Autodesk Fusion 360 part; units mm, degrees
(part 4 of 5)
sketch "Reset guide collar profile" plane through (0, 0, -12.5) normal (0, 0, 1) x (1, 0, 0) in component "05 Rear electronics housing"
  line L0 (116.2, 51) -> (117.8, 51)
  line L1 (117.8, 51) -> (117.8, 57.2)
  line L2 (117.8, 57.2) -> (116.2, 57.2)
  line L3 (116.2, 57.2) -> (116.2, 51)
  dimension "d865" = 1.6
  dimension "d866" = 6.2
  measures "d865" horizontal distance of L0.start L0.end
  measures "d866" vertical distance of L0.end L1.end
extrude "Reset guide collar" add sketch "Reset guide collar profile" against normal blind 5.3 separate body makes body 101 in component "05 Rear electronics housing"
ref_plane "WorkPlane58" through (0, 51, 0) normal (0, 1, 0) x (0, 0, 1) in component "05 Rear electronics housing"
sketch "Reset collar underside gusset" plane through (0, 51, 0) normal (0, 1, 0) x (1, 0, 0) in component "05 Rear electronics housing"
  line L0 (116.2, 17.8) -> (117.8, 17.8)
  line L1 (117.8, 17.8) -> (117.8, 19.4)
  line L2 (117.8, 19.4) -> (116.2, 17.8)
extrude "Reset collar underside gusset (1)" add sketch "Reset collar underside gusset" along normal blind 6.2 separate body makes body 102 in component "05 Rear electronics housing"
ref_plane "WorkPlane59" through (0, 0, -15.65) normal (0, 0, 1) x (1, 0, 0) in component "05 Rear electronics housing"
sketch "Reset stop root profile" plane through (0, 0, -15.65) normal (0, 0, 1) x (1, 0, 0) in component "05 Rear electronics housing"
  line L0 (114.2, 50.6) -> (117.8, 50.6)
  line L1 (117.8, 50.6) -> (117.8, 51.6)
  line L2 (117.8, 51.6) -> (114.2, 51.6)
  line L3 (114.2, 51.6) -> (114.2, 50.6)
  dimension "d875" = 3.6
  dimension "d876" = 1
  measures "d875" horizontal distance of L0.start L0.end
  measures "d876" vertical distance of L0.end L1.end
extrude "Reset stop root" add sketch "Reset stop root profile" against normal blind 1.75 separate body makes body 103 in component "05 Rear electronics housing"
ref_plane "WorkPlane60" through (0, 50.6, 0) normal (0, 1, 0) x (0, 0, 1) in component "05 Rear electronics housing"
sketch "Reset stop root gusset" plane through (0, 50.6, 0) normal (0, 1, 0) x (1, 0, 0) in component "05 Rear electronics housing"
  line L0 (114.2, 17.4) -> (117.8, 17.4)
  line L1 (117.8, 17.4) -> (117.8, 21)
  line L2 (117.8, 21) -> (114.2, 17.4)
extrude "Reset stop root gusset (1)" add sketch "Reset stop root gusset" along normal blind 1 separate body makes body 104 in component "05 Rear electronics housing"
ref_plane "WorkPlane61" through (0, 0, -15.65) normal (0, 0, 1) x (1, 0, 0) in component "05 Rear electronics housing"
sketch "Reset inward stop profile" plane through (0, 0, -15.65) normal (0, 0, 1) x (1, 0, 0) in component "05 Rear electronics housing"
  line L0 (114.2, 51.6) -> (114.7, 51.6)
  line L1 (114.7, 51.6) -> (114.7, 53.2)
  line L2 (114.7, 53.2) -> (114.2, 53.2)
  line L3 (114.2, 53.2) -> (114.2, 51.6)
  dimension "d885" = 0.5
  dimension "d886" = 1.6
  measures "d885" horizontal distance of L0.start L0.end
  measures "d886" vertical distance of L0.end L1.end
extrude "Reset inward stop" add sketch "Reset inward stop profile" against normal blind 1.75 separate body makes body 105 in component "05 Rear electronics housing"
combine "Union manufactured solid (8)" operation add target body 66 tool bodies 101 102 103 104 105 in component "05 Rear electronics housing"
ref_plane "WorkPlane62" through (0, 57.4, 0) normal (0, 1, 0) x (0, 0, 1) in component "05 Rear electronics housing"
sketch "Charger USB access" plane through (0, 57.4, 0) normal (0, 1, 0) x (1, 0, 0) in component "05 Rear electronics housing"
  line L0 (14.8, 26.2) -> (28.2, 26.2)
  line L1 (28.2, 26.2) -> (28.2, 20.5)
  line L2 (28.2, 20.5) -> (26.2, 18.5)
  line L3 (26.2, 18.5) -> (16.8, 18.5)
  line L4 (16.8, 18.5) -> (14.8, 20.5)
  line L5 (14.8, 20.5) -> (14.8, 26.2)
extrude "Charger USB access (1)" cut sketch "Charger USB access" along normal blind 2.8 bodies 66 in component "05 Rear electronics housing"
ref_plane "WorkPlane63" through (0, 57.4, 0) normal (0, 1, 0) x (0, 0, 1) in component "05 Rear electronics housing"
sketch "XIAO USB access" plane through (0, 57.4, 0) normal (0, 1, 0) x (1, 0, 0) in component "05 Rear electronics housing"
  line L0 (110.4, 28) -> (117.5, 28)
  line L1 (117.5, 28) -> (117.5, 18)
  line L2 (117.5, 18) -> (116, 16.5)
  line L3 (116, 16.5) -> (111.9, 16.5)
  line L4 (111.9, 16.5) -> (110.4, 18)
  line L5 (110.4, 18) -> (110.4, 28)
extrude "XIAO USB access (1)" cut sketch "XIAO USB access" along normal blind 2.8 bodies 66 in component "05 Rear electronics housing"
ref_plane "WorkPlane64" through (0, 57.4, 0) normal (0, 1, 0) x (0, 0, 1) in component "05 Rear electronics housing"
sketch "Power grip insertion and travel" plane through (0, 57.4, 0) normal (0, 1, 0) x (1, 0, 0) in component "05 Rear electronics housing"
  line L0 (55.25, 24.1) -> (64.75, 24.1)
  line L1 (64.75, 24.1) -> (64.75, 21.1)
  line L2 (64.75, 21.1) -> (62.75, 19.1)
  line L3 (62.75, 19.1) -> (57.25, 19.1)
  line L4 (57.25, 19.1) -> (55.25, 21.1)
  line L5 (55.25, 21.1) -> (55.25, 24.1)
extrude "Power grip insertion and travel (1)" cut sketch "Power grip insertion and travel" along normal blind 2.8 bodies 66 in component "05 Rear electronics housing"
ref_plane "WorkPlane65" through (116.1, 0, 0) normal (1, 0, 0) x (0, 1, 0) in component "05 Rear electronics housing"
sketch "Reset stem guide" plane through (116.1, 0, 0) normal (1, 0, 0) x (0, 0, -1) in component "05 Rear electronics housing"
  line L0 (16.6, 52.55) -> (16.6, 56.85)
  line L1 (16.6, 56.85) -> (14, 56.85)
  line L2 (14, 56.85) -> (13.7, 56.55)
  line L3 (13.7, 56.55) -> (13.7, 52.85)
  line L4 (13.7, 52.85) -> (14, 52.55)
  line L5 (14, 52.55) -> (16.6, 52.55)
extrude "Reset stem guide (1)" cut sketch "Reset stem guide" along normal blind 4.1 bodies 66 in component "05 Rear electronics housing"
ref_plane "WorkPlane66" through (0, 0, -15.64) normal (0, 0, 1) x (1, 0, 0) in component "05 Rear electronics housing"
sketch "Open reset insertion path - stop moved to yoke profile" plane through (0, 0, -15.64) normal (0, 0, 1) x (1, 0, 0) in component "05 Rear electronics housing"
  line L0 (114.19, 50.59) -> (116.19, 50.59)
  line L1 (116.19, 50.59) -> (116.19, 53.21)
  line L2 (116.19, 53.21) -> (114.19, 53.21)
  line L3 (114.19, 53.21) -> (114.19, 50.59)
  dimension "d907" = 2
  dimension "d908" = 2.62
  measures "d907" horizontal distance of L0.start L0.end
  measures "d908" vertical distance of L0.end L1.end
extrude "Open reset insertion path - stop moved to yoke" cut sketch "Open reset insertion path - stop moved to yoke profile" against normal blind 5.37 bodies 66 in component "05 Rear electronics housing"
ref_plane "WorkPlane1" through (0, 0, -9.4) normal (0, 0, 1) x (1, 0, 0) in component "06 Electronics retaining yoke"
sketch "Common yoke rail profile" plane through (0, 0, -9.4) normal (0, 0, 1) x (1, 0, 0) in component "06 Electronics retaining yoke"
  line L0 (11.1, 36) -> (112.3, 36)
  line L1 (112.3, 36) -> (112.3, 39)
  line L2 (112.3, 39) -> (11.1, 39)
  line L3 (11.1, 39) -> (11.1, 36)
  dimension "d913" = 101.2
  dimension "d914" = 3
  measures "d913" horizontal distance of L0.start L0.end
  measures "d914" vertical distance of L0.end L1.end
extrude "Common yoke rail" add sketch "Common yoke rail profile" against normal blind 2 separate body makes body 106 in component "06 Electronics retaining yoke"
ref_plane "WorkPlane2" through (0, 0, -9.4) normal (0, 0, 1) x (1, 0, 0) in component "06 Electronics retaining yoke"
sketch "Charger yoke arm profile" plane through (0, 0, -9.4) normal (0, 0, 1) x (1, 0, 0) in component "06 Electronics retaining yoke"
  line L0 (11.1, 34) -> (15.7, 34)
  line L1 (15.7, 34) -> (15.7, 53)
  line L2 (15.7, 53) -> (11.1, 53)
  line L3 (11.1, 53) -> (11.1, 34)
  dimension "d919" = 4.6
  dimension "d920" = 19
  measures "d919" horizontal distance of L0.start L0.end
  measures "d920" vertical distance of L0.end L1.end
extrude "Charger yoke arm" add sketch "Charger yoke arm profile" against normal blind 2 separate body makes body 107 in component "06 Electronics retaining yoke"
ref_plane "WorkPlane3" through (0, 0, -9.4) normal (0, 0, 1) x (1, 0, 0) in component "06 Electronics retaining yoke"
sketch "Charger yoke arm profile (1)" plane through (0, 0, -9.4) normal (0, 0, 1) x (1, 0, 0) in component "06 Electronics retaining yoke"
  line L0 (26.9, 34) -> (31.5, 34)
  line L1 (31.5, 34) -> (31.5, 53)
  line L2 (31.5, 53) -> (26.9, 53)
  line L3 (26.9, 53) -> (26.9, 34)
  dimension "d925" = 4.6
  dimension "d926" = 19
  measures "d925" horizontal distance of L0.start L0.end
  measures "d926" vertical distance of L0.end L1.end
extrude "Charger yoke arm (1)" add sketch "Charger yoke arm profile (1)" against normal blind 2 separate body makes body 108 in component "06 Electronics retaining yoke"
ref_plane "WorkPlane4" through (0, 0, -11.4) normal (0, 0, 1) x (1, 0, 0) in component "06 Electronics retaining yoke"
sketch "Charger keeper foot profile" plane through (0, 0, -11.4) normal (0, 0, 1) x (1, 0, 0) in component "06 Electronics retaining yoke"
  line L0 (13.1, 34) -> (15.1, 34)
  line L1 (15.1, 34) -> (15.1, 36)
  line L2 (15.1, 36) -> (13.1, 36)
  line L3 (13.1, 36) -> (13.1, 34)
  dimension "d931" = 2
  dimension "d932" = 2
  measures "d931" horizontal distance of L0.start L0.end
  measures "d932" vertical distance of L0.end L1.end
extrude "Charger keeper foot" add sketch "Charger keeper foot profile" against normal blind 11.65 separate body makes body 109 in component "06 Electronics retaining yoke"
ref_plane "WorkPlane5" through (0, 0, -11.4) normal (0, 0, 1) x (1, 0, 0) in component "06 Electronics retaining yoke"
sketch "Charger keeper foot profile (1)" plane through (0, 0, -11.4) normal (0, 0, 1) x (1, 0, 0) in component "06 Electronics retaining yoke"
  line L0 (26.9, 34) -> (28.9, 34)
  line L1 (28.9, 34) -> (28.9, 36)
  line L2 (28.9, 36) -> (26.9, 36)
  line L3 (26.9, 36) -> (26.9, 34)
  dimension "d937" = 2
  dimension "d938" = 2
  measures "d937" horizontal distance of L0.start L0.end
  measures "d938" vertical distance of L0.end L1.end
extrude "Charger keeper foot (1)" add sketch "Charger keeper foot profile (1)" against normal blind 11.65 separate body makes body 110 in component "06 Electronics retaining yoke"
ref_plane "WorkPlane6" through (0, 0, -11.4) normal (0, 0, 1) x (1, 0, 0) in component "06 Electronics retaining yoke"
sketch "Charger keeper foot profile (2)" plane through (0, 0, -11.4) normal (0, 0, 1) x (1, 0, 0) in component "06 Electronics retaining yoke"
  line L0 (13.1, 51) -> (15.1, 51)
  line L1 (15.1, 51) -> (15.1, 53)
  line L2 (15.1, 53) -> (13.1, 53)
  line L3 (13.1, 53) -> (13.1, 51)
  dimension "d943" = 2
  dimension "d944" = 2
  measures "d943" horizontal distance of L0.start L0.end
  measures "d944" vertical distance of L0.end L1.end
extrude "Charger keeper foot (2)" add sketch "Charger keeper foot profile (2)" against normal blind 11.65 separate body makes body 111 in component "06 Electronics retaining yoke"
ref_plane "WorkPlane7" through (0, 0, -11.4) normal (0, 0, 1) x (1, 0, 0) in component "06 Electronics retaining yoke"
sketch "Charger keeper foot profile (3)" plane through (0, 0, -11.4) normal (0, 0, 1) x (1, 0, 0) in component "06 Electronics retaining yoke"
  line L0 (26.9, 51) -> (28.9, 51)
  line L1 (28.9, 51) -> (28.9, 53)
  line L2 (28.9, 53) -> (26.9, 53)
  line L3 (26.9, 53) -> (26.9, 51)
  dimension "d949" = 2
  dimension "d950" = 2
  measures "d949" horizontal distance of L0.start L0.end
  measures "d950" vertical distance of L0.end L1.end
extrude "Charger keeper foot (3)" add sketch "Charger keeper foot profile (3)" against normal blind 11.65 separate body makes body 112 in component "06 Electronics retaining yoke"
ref_plane "WorkPlane8" through (0, 0, -9.4) normal (0, 0, 1) x (1, 0, 0) in component "06 Electronics retaining yoke"
sketch "Switch yoke arm profile" plane through (0, 0, -9.4) normal (0, 0, 1) x (1, 0, 0) in component "06 Electronics retaining yoke"
  line L0 (53.5, 37) -> (56.9, 37)
  line L1 (56.9, 37) -> (56.9, 52)
  line L2 (56.9, 52) -> (53.5, 52)
  line L3 (53.5, 52) -> (53.5, 37)
  dimension "d955" = 3.4
  dimension "d956" = 15
  measures "d955" horizontal distance of L0.start L0.end
  measures "d956" vertical distance of L0.end L1.end
extrude "Switch yoke arm" add sketch "Switch yoke arm profile" against normal blind 2 separate body makes body 113 in component "06 Electronics retaining yoke"
ref_plane "WorkPlane9" through (0, 0, -9.4) normal (0, 0, 1) x (1, 0, 0) in component "06 Electronics retaining yoke"
sketch "Switch yoke arm profile (1)" plane through (0, 0, -9.4) normal (0, 0, 1) x (1, 0, 0) in component "06 Electronics retaining yoke"
  line L0 (63.1, 37) -> (66.5, 37)
  line L1 (66.5, 37) -> (66.5, 52)
  line L2 (66.5, 52) -> (63.1, 52)
  line L3 (63.1, 52) -> (63.1, 37)
  dimension "d961" = 3.4
  dimension "d962" = 15
  measures "d961" horizontal distance of L0.start L0.end
  measures "d962" vertical distance of L0.end L1.end
extrude "Switch yoke arm (1)" add sketch "Switch yoke arm profile (1)" against normal blind 2 separate body makes body 114 in component "06 Electronics retaining yoke"
ref_plane "WorkPlane10" through (0, 0, -11.4) normal (0, 0, 1) x (1, 0, 0) in component "06 Electronics retaining yoke"
sketch "Switch retaining foot profile" plane through (0, 0, -11.4) normal (0, 0, 1) x (1, 0, 0) in component "06 Electronics retaining yoke"
  line L0 (55.9, 49.7) -> (56.9, 49.7)
  line L1 (56.9, 49.7) -> (56.9, 52)
  line L2 (56.9, 52) -> (55.9, 52)
  line L3 (55.9, 52) -> (55.9, 49.7)
  dimension "d967" = 1
  dimension "d968" = 2.3
  measures "d967" horizontal distance of L0.start L0.end
  measures "d968" vertical distance of L0.end L1.end
extrude "Switch retaining foot" add sketch "Switch retaining foot profile" against normal blind 8.45 separate body makes body 115 in component "06 Electronics retaining yoke"
ref_plane "WorkPlane11" through (0, 0, -11.4) normal (0, 0, 1) x (1, 0, 0) in component "06 Electronics retaining yoke"
sketch "Switch retaining foot profile (1)" plane through (0, 0, -11.4) normal (0, 0, 1) x (1, 0, 0) in component "06 Electronics retaining yoke"
  line L0 (63.1, 49.7) -> (64.1, 49.7)
  line L1 (64.1, 49.7) -> (64.1, 52)
  line L2 (64.1, 52) -> (63.1, 52)
  line L3 (63.1, 52) -> (63.1, 49.7)
  dimension "d973" = 1
  dimension "d974" = 2.3
  measures "d973" horizontal distance of L0.start L0.end
  measures "d974" vertical distance of L0.end L1.end
extrude "Switch retaining foot (1)" add sketch "Switch retaining foot profile (1)" against normal blind 8.45 separate body makes body 116 in component "06 Electronics retaining yoke"
ref_plane "WorkPlane12" through (0, 0, -9.4) normal (0, 0, 1) x (1, 0, 0) in component "06 Electronics retaining yoke"
sketch "XIAO yoke rail profile" plane through (0, 0, -9.4) normal (0, 0, 1) x (1, 0, 0) in component "06 Electronics retaining yoke"
  line L0 (108.5, 38) -> (112.3, 38)
  line L1 (112.3, 38) -> (112.3, 50)
  line L2 (112.3, 50) -> (108.5, 50)
  line L3 (108.5, 50) -> (108.5, 38)
  dimension "d979" = 3.8
  dimension "d980" = 12
  measures "d979" horizontal distance of L0.start L0.end
  measures "d980" vertical distance of L0.end L1.end
extrude "XIAO yoke rail" add sketch "XIAO yoke rail profile" against normal blind 2 separate body makes body 117 in component "06 Electronics retaining yoke"
ref_plane "WorkPlane13" through (0, 0, -9.4) normal (0, 0, 1) x (1, 0, 0) in component "06 Electronics retaining yoke"
sketch "Reset stop arm profile" plane through (0, 0, -9.4) normal (0, 0, 1) x (1, 0, 0) in component "06 Electronics retaining yoke"
  line L0 (108.5, 49) -> (115.4, 49)
  line L1 (115.4, 49) -> (115.4, 51.6)
  line L2 (115.4, 51.6) -> (108.5, 51.6)
  line L3 (108.5, 51.6) -> (108.5, 49)
  dimension "d985" = 6.9
  dimension "d986" = 2.6
  measures "d985" horizontal distance of L0.start L0.end
  measures "d986" vertical distance of L0.end L1.end
extrude "Reset stop arm" add sketch "Reset stop arm profile" against normal blind 2 separate body makes body 118 in component "06 Electronics retaining yoke"
ref_plane "WorkPlane14" through (0, 0, -11.4) normal (0, 0, 1) x (1, 0, 0) in component "06 Electronics retaining yoke"
sketch "Reset stop post profile" plane through (0, 0, -11.4) normal (0, 0, 1) x (1, 0, 0) in component "06 Electronics retaining yoke"
  line L0 (113.5, 50.6) -> (115.4, 50.6)
  line L1 (115.4, 50.6) -> (115.4, 51.6)
  line L2 (115.4, 51.6) -> (113.5, 51.6)
  line L3 (113.5, 51.6) -> (113.5, 50.6)
  dimension "d991" = 1.9
  dimension "d992" = 1
  measures "d991" horizontal distance of L0.start L0.end
  measures "d992" vertical distance of L0.end L1.end
extrude "Reset stop post" add sketch "Reset stop post profile" against normal blind 6 separate body makes body 119 in component "06 Electronics retaining yoke"
ref_plane "WorkPlane15" through (0, 0, -15.65) normal (0, 0, 1) x (1, 0, 0) in component "06 Electronics retaining yoke"
sketch "Reset inward stop profile (2)" plane through (0, 0, -15.65) normal (0, 0, 1) x (1, 0, 0) in component "06 Electronics retaining yoke"
  line L0 (113.5, 51.6) -> (114.7, 51.6)
  line L1 (114.7, 51.6) -> (114.7, 53.2)
  line L2 (114.7, 53.2) -> (113.5, 53.2)
  line L3 (113.5, 53.2) -> (113.5, 51.6)
  dimension "d997" = 1.2
  dimension "d998" = 1.6
  measures "d997" horizontal distance of L0.start L0.end
  measures "d998" vertical distance of L0.end L1.end
extrude "Reset inward stop'" add sketch "Reset inward stop profile (2)" against normal blind 1.75 separate body makes body 120 in component "06 Electronics retaining yoke"
ref_plane "WorkPlane16" through (113.5, 0, 0) normal (1, 0, 0) x (0, 1, 0) in component "06 Electronics retaining yoke"
sketch "Reset stop 45 degree brace" plane through (113.5, 0, 0) normal (1, 0, 0) x (0, 0, -1) in component "06 Electronics retaining yoke"
  line L0 (14.05, 51.6) -> (15.65, 51.6)
  line L1 (15.65, 51.6) -> (15.65, 53.2)
  line L2 (15.65, 53.2) -> (14.05, 51.6)
extrude "Reset stop 45 degree brace (1)" add sketch "Reset stop 45 degree brace" along normal blind 1.2 separate body makes body 121 in component "06 Electronics retaining yoke"
ref_plane "WorkPlane17" through (0, 0, -9.4) normal (0, 0, 1) x (1, 0, 0) in component "06 Electronics retaining yoke"
sketch "XIAO restraint root profile" plane through (0, 0, -9.4) normal (0, 0, 1) x (1, 0, 0) in component "06 Electronics retaining yoke"
  line L0 (111.8, 40) -> (113.75, 40)
  line L1 (113.75, 40) -> (113.75, 42)
  line L2 (113.75, 42) -> (111.8, 42)
  line L3 (111.8, 42) -> (111.8, 40)
  dimension "d1007" = 1.95
  dimension "d1008" = 2
  measures "d1007" horizontal distance of L0.start L0.end
  measures "d1008" vertical distance of L0.end L1.end
extrude "XIAO restraint root" add sketch "XIAO restraint root profile" against normal blind 2 separate body makes body 122 in component "06 Electronics retaining yoke"
ref_plane "WorkPlane18" through (0, 0, -11.3) normal (0, 0, 1) x (1, 0, 0) in component "06 Electronics retaining yoke"
sketch "XIAO front outer restraint profile" plane through (0, 0, -11.3) normal (0, 0, 1) x (1, 0, 0) in component "06 Electronics retaining yoke"
  line L0 (112.25, 40) -> (113.75, 40)
  line L1 (113.75, 40) -> (113.75, 42)
  line L2 (113.75, 42) -> (112.25, 42)
  line L3 (112.25, 42) -> (112.25, 40)
  dimension "d1013" = 1.5
  dimension "d1014" = 2
  measures "d1013" horizontal distance of L0.start L0.end
  measures "d1014" vertical distance of L0.end L1.end
extrude "XIAO front outer restraint" add sketch "XIAO front outer restraint profile" against normal blind 2.4 separate body makes body 123 in component "06 Electronics retaining yoke"
ref_plane "WorkPlane19" through (0, 0, -9.4) normal (0, 0, 1) x (1, 0, 0) in component "06 Electronics retaining yoke"
sketch "XIAO restraint root profile (1)" plane through (0, 0, -9.4) normal (0, 0, 1) x (1, 0, 0) in component "06 Electronics retaining yoke"
  line L0 (111.8, 48) -> (113.75, 48)
  line L1 (113.75, 48) -> (113.75, 50)
  line L2 (113.75, 50) -> (111.8, 50)
  line L3 (111.8, 50) -> (111.8, 48)
  dimension "d1019" = 1.95
  dimension "d1020" = 2
  measures "d1019" horizontal distance of L0.start L0.end
  measures "d1020" vertical distance of L0.end L1.end
extrude "XIAO restraint root (1)" add sketch "XIAO restraint root profile (1)" against normal blind 2 separate body makes body 124 in component "06 Electronics retaining yoke"
ref_plane "WorkPlane20" through (0, 0, -11.3) normal (0, 0, 1) x (1, 0, 0) in component "06 Electronics retaining yoke"
sketch "XIAO front outer restraint profile (1)" plane through (0, 0, -11.3) normal (0, 0, 1) x (1, 0, 0) in component "06 Electronics retaining yoke"
  line L0 (112.25, 48) -> (113.75, 48)
  line L1 (113.75, 48) -> (113.75, 50)
  line L2 (113.75, 50) -> (112.25, 50)
  line L3 (112.25, 50) -> (112.25, 48)
  dimension "d1025" = 1.5
  dimension "d1026" = 2
  measures "d1025" horizontal distance of L0.start L0.end
  measures "d1026" vertical distance of L0.end L1.end
extrude "XIAO front outer restraint (1)" add sketch "XIAO front outer restraint profile (1)" against normal blind 2.4 separate body makes body 125 in component "06 Electronics retaining yoke"
ref_plane "WorkPlane21" through (0, 0, -9.4) normal (0, 0, 1) x (1, 0, 0) in component "06 Electronics retaining yoke"
sketch "Yoke screw pad profile" plane through (0, 0, -9.4) normal (0, 0, 1) x (1, 0, 0) in component "06 Electronics retaining yoke"
  line L0 (30.8, 33.8) -> (39.2, 33.8)
  line L1 (39.2, 33.8) -> (39.2, 42.2)
  line L2 (39.2, 42.2) -> (30.8, 42.2)
  line L3 (30.8, 42.2) -> (30.8, 33.8)
  dimension "d1031" = 8.4
  dimension "d1032" = 8.4
  measures "d1031" horizontal distance of L0.start L0.end
  measures "d1032" vertical distance of L0.end L1.end
extrude "Yoke screw pad" add sketch "Yoke screw pad profile" against normal blind 2 separate body makes body 126 in component "06 Electronics retaining yoke"
ref_plane "WorkPlane22" through (0, 0, -9.4) normal (0, 0, 1) x (1, 0, 0) in component "06 Electronics retaining yoke"
sketch "Yoke screw pad profile (1)" plane through (0, 0, -9.4) normal (0, 0, 1) x (1, 0, 0) in component "06 Electronics retaining yoke"
  line L0 (98.8, 33.8) -> (107.2, 33.8)
  line L1 (107.2, 33.8) -> (107.2, 42.2)
  line L2 (107.2, 42.2) -> (98.8, 42.2)
  line L3 (98.8, 42.2) -> (98.8, 33.8)
  dimension "d1037" = 8.4
  dimension "d1038" = 8.4
  measures "d1037" horizontal distance of L0.start L0.end
  measures "d1038" vertical distance of L0.end L1.end
extrude "Yoke screw pad (1)" add sketch "Yoke screw pad profile (1)" against normal blind 2 separate body makes body 127 in component "06 Electronics retaining yoke"
combine "Union manufactured solid''''" operation add target body 106 tool bodies 107 108 109 110 111 112 113 114 115 116 117 118 119 120 121 122 123 124 125 126 127 in component "06 Electronics retaining yoke"
ref_plane "WorkPlane23" through (0, 0, -9.38) normal (0, 0, 1) x (1, 0, 0) in component "06 Electronics retaining yoke"
sketch "Yoke M3 clearance profile" plane through (0, 0, -9.38) normal (0, 0, 1) x (1, 0, 0) in component "06 Electronics retaining yoke"
  circle A0 centre (35, 38) radius 1.7
  dimension "d1043" = 3.4
  measures "d1043" diameter of A0
extrude "Yoke M3 clearance" cut sketch "Yoke M3 clearance profile" against normal blind 2.04 bodies 106 in component "06 Electronics retaining yoke"
ref_plane "WorkPlane24" through (0, 0, -9.38) normal (0, 0, 1) x (1, 0, 0) in component "06 Electronics retaining yoke"
sketch "Yoke M3 clearance profile (1)" plane through (0, 0, -9.38) normal (0, 0, 1) x (1, 0, 0) in component "06 Electronics retaining yoke"
  circle A0 centre (103, 38) radius 1.7
  dimension "d1048" = 3.4
  measures "d1048" diameter of A0
extrude "Yoke M3 clearance (1)" cut sketch "Yoke M3 clearance profile (1)" against normal blind 2.04 bodies 106 in component "06 Electronics retaining yoke"
ref_plane "WorkPlane1" through (0, 0, -13.95) normal (0, 0, 1) x (1, 0, 0) in component "07 Captive reset plunger"
sketch "Reset exterior stem profile" plane through (0, 0, -13.95) normal (0, 0, 1) x (1, 0, 0) in component "07 Captive reset plunger"
  line L0 (116, 52.8) -> (120.6, 52.8)
  line L1 (120.6, 52.8) -> (120.6, 56.6)
  line L2 (120.6, 56.6) -> (116, 56.6)
  line L3 (116, 56.6) -> (116, 52.8)
  dimension "d1053" = 4.6
  dimension "d1054" = 3.8
  measures "d1053" horizontal distance of L0.start L0.end
  measures "d1054" vertical distance of L0.end L1.end
extrude "Reset exterior stem" add sketch "Reset exterior stem profile" against normal blind 2.4 separate body makes body 128 in component "07 Captive reset plunger"
ref_plane "WorkPlane2" through (0, 0, -13.95) normal (0, 0, 1) x (1, 0, 0) in component "07 Captive reset plunger"
sketch "Reset captive flange profile" plane through (0, 0, -13.95) normal (0, 0, 1) x (1, 0, 0) in component "07 Captive reset plunger"
  line L0 (115.2, 51.9) -> (116, 51.9)
  line L1 (116, 51.9) -> (116, 57.5)
  line L2 (116, 57.5) -> (115.2, 57.5)
  line L3 (115.2, 57.5) -> (115.2, 51.9)
  dimension "d1059" = 0.8
  dimension "d1060" = 5.6
  measures "d1059" horizontal distance of L0.start L0.end
  measures "d1060" vertical distance of L0.end L1.end
extrude "Reset captive flange" add sketch "Reset captive flange profile" against normal blind 3.2 separate body makes body 129 in component "07 Captive reset plunger"
ref_plane "WorkPlane3" through (0, 0, -13.95) normal (0, 0, 1) x (1, 0, 0) in component "07 Captive reset plunger"
sketch "Reset contact tip profile" plane through (0, 0, -13.95) normal (0, 0, 1) x (1, 0, 0) in component "07 Captive reset plunger"
  line L0 (113.7, 53.9) -> (115.2, 53.9)
  line L1 (115.2, 53.9) -> (115.2, 55.5)
  line L2 (115.2, 55.5) -> (113.7, 55.5)
  line L3 (113.7, 55.5) -> (113.7, 53.9)
  dimension "d1065" = 1.5
  dimension "d1066" = 1.6
  measures "d1065" horizontal distance of L0.start L0.end
  measures "d1066" vertical distance of L0.end L1.end
extrude "Reset contact tip" add sketch "Reset contact tip profile" against normal blind 1.2 separate body makes body 130 in component "07 Captive reset plunger"
combine "Union manufactured solid'''''" operation add target body 128 tool bodies 129 130 in component "07 Captive reset plunger"
ref_plane "WorkPlane1" through (0, 0, -20.05) normal (0, 0, 1) x (1, 0, 0) in component "08 Captive DPDT power slider"
sketch "Actuator cup blank profile" plane through (0, 0, -20.05) normal (0, 0, 1) x (1, 0, 0) in component "08 Captive DPDT power slider"
  line L0 (57.7, 52.4) -> (62.3, 52.4)
  line L1 (62.3, 52.4) -> (62.3, 53.4)
  line L2 (62.3, 53.4) -> (57.7, 53.4)
  line L3 (57.7, 53.4) -> (57.7, 52.4)
  dimension "d1071" = 4.6
  dimension "d1072" = 1
  measures "d1071" horizontal distance of L0.start L0.end
  measures "d1072" vertical distance of L0.end L1.end
extrude "Actuator cup blank" add sketch "Actuator cup blank profile" against normal blind 3.3 separate body makes body 131 in component "08 Captive DPDT power slider"
ref_plane "WorkPlane2" through (0, 53.4, 0) normal (0, 1, 0) x (0, 0, 1) in component "08 Captive DPDT power slider"
sketch "Slider shoulder lower" plane through (0, 53.4, 0) normal (0, 1, 0) x (1, 0, 0) in component "08 Captive DPDT power slider"
  line L0 (57.7, 20.05) -> (62.3, 20.05)
  line L1 (62.3, 20.05) -> (62.3, 23.35)
  line L2 (62.3, 23.35) -> (57.7, 23.35)
  line L3 (57.7, 23.35) -> (57.7, 20.05)
ref_plane "WorkPlane3" through (0, 57.1, 0) normal (0, 1, 0) x (0, 0, 1) in component "08 Captive DPDT power slider"
sketch "Slider shoulder upper" plane through (0, 57.1, 0) normal (0, 1, 0) x (1, 0, 0) in component "08 Captive DPDT power slider"
  line L0 (54, 18.5) -> (66, 18.5)
  line L1 (66, 18.5) -> (66, 25.5)
  line L2 (66, 25.5) -> (54, 25.5)
  line L3 (54, 25.5) -> (54, 18.5)
loft "Self-supporting slider shoulder" add profiles "Slider shoulder lower", "Slider shoulder upper" section 1 section 2 separate body makes body 132 in component "08 Captive DPDT power slider"
ref_plane "WorkPlane4" through (0, 0, -18.5) normal (0, 0, 1) x (1, 0, 0) in component "08 Captive DPDT power slider"
sketch "Inner captive flange profile" plane through (0, 0, -18.5) normal (0, 0, 1) x (1, 0, 0) in component "08 Captive DPDT power slider"
  line L0 (54, 57.05) -> (66, 57.05)
  line L1 (66, 57.05) -> (66, 57.4)
  line L2 (66, 57.4) -> (54, 57.4)
  line L3 (54, 57.4) -> (54, 57.05)
  dimension "d1081" = 12
  dimension "d1082" = 0.35
  measures "d1081" horizontal distance of L0.start L0.end
  measures "d1082" vertical distance of L0.end L1.end
extrude "Inner captive flange" add sketch "Inner captive flange profile" against normal blind 7 separate body makes body 133 in component "08 Captive DPDT power slider"
ref_plane "WorkPlane5" through (0, 0, -20.8) normal (0, 0, 1) x (1, 0, 0) in component "08 Captive DPDT power slider"
sketch "Slider guide neck profile" plane through (0, 0, -20.8) normal (0, 0, 1) x (1, 0, 0) in component "08 Captive DPDT power slider"
  line L0 (57.6, 57.3) -> (62.4, 57.3)
  line L1 (62.4, 57.3) -> (62.4, 60.8)
  line L2 (62.4, 60.8) -> (57.6, 60.8)
  line L3 (57.6, 60.8) -> (57.6, 57.3)
  dimension "d1087" = 4.8
  dimension "d1088" = 3.5
  measures "d1087" horizontal distance of L0.start L0.end
  measures "d1088" vertical distance of L0.end L1.end
extrude "Slider guide neck" add sketch "Slider guide neck profile" against normal blind 2.4 separate body makes body 134 in component "08 Captive DPDT power slider"
ref_plane "WorkPlane6" through (0, 0, -20.6) normal (0, 0, 1) x (1, 0, 0) in component "08 Captive DPDT power slider"
sketch "Exterior finger grip profile" plane through (0, 0, -20.6) normal (0, 0, 1) x (1, 0, 0) in component "08 Captive DPDT power slider"
  line L0 (57.5, 60) -> (62.5, 60)
  line L1 (62.5, 60) -> (62.5, 61.4)
  line L2 (62.5, 61.4) -> (57.5, 61.4)
  line L3 (57.5, 61.4) -> (57.5, 60)
  dimension "d1093" = 5
  dimension "d1094" = 1.4
  measures "d1093" horizontal distance of L0.start L0.end
  measures "d1094" vertical distance of L0.end L1.end
extrude "Exterior finger grip" add sketch "Exterior finger grip profile" against normal blind 2.8 separate body makes body 135 in component "08 Captive DPDT power slider"
combine "Union manufactured solid''''''" operation add target body 131 tool bodies 132 133 134 135 in component "08 Captive DPDT power slider"
ref_plane "WorkPlane7" through (0, 0, -18) normal (0, 0, 1) x (1, 0, 0) in component "08 Captive DPDT power slider"
sketch "Front and bottom open actuator fork profile" plane through (0, 0, -18) normal (0, 0, 1) x (1, 0, 0) in component "08 Captive DPDT power slider"
  line L0 (59.09, 52.3) -> (60.91, 52.3)
  line L1 (60.91, 52.3) -> (60.91, 54.43)
  line L2 (60.91, 54.43) -> (59.09, 54.43)
  line L3 (59.09, 54.43) -> (59.09, 52.3)
  dimension "d1099" = 1.82
  dimension "d1100" = 2.13
  measures "d1099" horizontal distance of L0.start L0.end
  measures "d1100" vertical distance of L0.end L1.end
extrude "Front and bottom open actuator fork" cut sketch "Front and bottom open actuator fork profile" against normal blind 4.46 bodies 131 in component "08 Captive DPDT power slider"
ref_plane "WorkPlane1" through (0, 0, -20.6) normal (0, 0, 1) x (1, 0, 0) in component "REF Battery"
sketch "Battery pouch profile" plane through (0, 0, -20.6) normal (0, 0, 1) x (1, 0, 0) in component "REF Battery"
  line L0 (35, 11) -> (87, 11)
  line L1 (87, 11) -> (87, 32)
  line L2 (87, 32) -> (35, 32)
  line L3 (35, 32) -> (35, 11)
  dimension "d1105" = 52
  dimension "d1106" = 21
  measures "d1105" horizontal distance of L0.start L0.end
  measures "d1106" vertical distance of L0.end L1.end
extrude "Battery pouch" add sketch "Battery pouch profile" against normal blind 10 separate body makes body 136 in component "REF Battery"
ref_plane "WorkPlane1" through (0, 0, -23.2) normal (0, 0, 1) x (1, 0, 0) in component "REF Charger"
sketch "Charger PCB profile" plane through (0, 0, -23.2) normal (0, 0, 1) x (1, 0, 0) in component "REF Charger"
  line L0 (12.75, 32) -> (29.25, 32)
  line L1 (29.25, 32) -> (29.25, 57)
  line L2 (29.25, 57) -> (12.75, 57)
  line L3 (12.75, 57) -> (12.75, 32)
  dimension "d1111" = 16.5
  dimension "d1112" = 25
  measures "d1111" horizontal distance of L0.start L0.end
  measures "d1112" vertical distance of L0.end L1.end
extrude "Charger PCB" add sketch "Charger PCB profile" against normal blind 1 separate body makes body 137 in component "REF Charger"
ref_plane "WorkPlane2" through (0, 0, -19.6) normal (0, 0, 1) x (1, 0, 0) in component "REF Charger"
sketch "Charger USB envelope profile" plane through (0, 0, -19.6) normal (0, 0, 1) x (1, 0, 0) in component "REF Charger"
  line L0 (17, 53) -> (26, 53)
  line L1 (26, 53) -> (26, 59.4)
  line L2 (26, 59.4) -> (17, 59.4)
  line L3 (17, 59.4) -> (17, 53)
  dimension "d1117" = 9
  dimension "d1118" = 6.4
  measures "d1117" horizontal distance of L0.start L0.end
  measures "d1118" vertical distance of L0.end L1.end
extrude "Charger USB envelope" add sketch "Charger USB envelope profile" against normal blind 3.6 separate body makes body 138 in component "REF Charger"
ref_plane "WorkPlane3" through (0, 0, -20.9) normal (0, 0, 1) x (1, 0, 0) in component "REF Charger"
sketch "Charger IC envelope profile" plane through (0, 0, -20.9) normal (0, 0, 1) x (1, 0, 0) in component "REF Charger"
  line L0 (18, 36) -> (25, 36)
  line L1 (25, 36) -> (25, 47)
  line L2 (25, 47) -> (18, 47)
  line L3 (18, 47) -> (18, 36)
  dimension "d1123" = 7
  dimension "d1124" = 11
  measures "d1123" horizontal distance of L0.start L0.end
  measures "d1124" vertical distance of L0.end L1.end
extrude "Charger IC envelope" add sketch "Charger IC envelope profile" against normal blind 2.3 separate body makes body 139 in component "REF Charger"
ref_plane "WorkPlane1" through (0, 0, -11.55) normal (0, 0, 1) x (1, 0, 0) in component "REF XIAO"
sketch "XIAO PCB profile" plane through (0, 0, -11.55) normal (0, 0, 1) x (1, 0, 0) in component "REF XIAO"
  line L0 (111, 35.5) -> (112, 35.5)
  line L1 (112, 35.5) -> (112, 56.5)
  line L2 (112, 56.5) -> (111, 56.5)
  line L3 (111, 56.5) -> (111, 35.5)
  dimension "d1129" = 1
  dimension "d1130" = 21
  measures "d1129" horizontal distance of L0.start L0.end
  measures "d1130" vertical distance of L0.end L1.end
extrude "XIAO PCB" add sketch "XIAO PCB profile" against normal blind 17.8 separate body makes body 140 in component "REF XIAO"
ref_plane "WorkPlane2" through (0, 0, -17.75) normal (0, 0, 1) x (1, 0, 0) in component "REF XIAO"
sketch "XIAO USB envelope profile" plane through (0, 0, -17.75) normal (0, 0, 1) x (1, 0, 0) in component "REF XIAO"
  line L0 (112, 52) -> (115.3, 52)
  line L1 (115.3, 52) -> (115.3, 58.4)
  line L2 (115.3, 58.4) -> (112, 58.4)
  line L3 (112, 58.4) -> (112, 52)
  dimension "d1135" = 3.3
  dimension "d1136" = 6.4
  measures "d1135" horizontal distance of L0.start L0.end
  measures "d1136" vertical distance of L0.end L1.end
extrude "XIAO USB envelope" add sketch "XIAO USB envelope profile" against normal blind 9 separate body makes body 141 in component "REF XIAO"
ref_plane "WorkPlane3" through (0, 0, -16) normal (0, 0, 1) x (1, 0, 0) in component "REF XIAO"
sketch "XIAO component envelope profile" plane through (0, 0, -16) normal (0, 0, 1) x (1, 0, 0) in component "REF XIAO"
  line L0 (112, 41.5) -> (115, 41.5)
  line L1 (115, 41.5) -> (115, 50.5)
  line L2 (115, 50.5) -> (112, 50.5)
  line L3 (112, 50.5) -> (112, 41.5)
  dimension "d1141" = 3
  dimension "d1142" = 9
  measures "d1141" horizontal distance of L0.start L0.end
  measures "d1142" vertical distance of L0.end L1.end
extrude "XIAO component envelope" add sketch "XIAO component envelope profile" against normal blind 9 separate body makes body 142 in component "REF XIAO"
ref_plane "WorkPlane4" through (0, 0, -13.65) normal (0, 0, 1) x (1, 0, 0) in component "REF XIAO"
sketch "XIAO reset target profile" plane through (0, 0, -13.65) normal (0, 0, 1) x (1, 0, 0) in component "REF XIAO"
  line L0 (112, 53.7) -> (113.5, 53.7)
  line L1 (113.5, 53.7) -> (113.5, 55.7)
  line L2 (113.5, 55.7) -> (112, 55.7)
  line L3 (112, 55.7) -> (112, 53.7)
  dimension "d1147" = 1.5
  dimension "d1148" = 2
  measures "d1147" horizontal distance of L0.start L0.end
  measures "d1148" vertical distance of L0.end L1.end
extrude "XIAO reset target" add sketch "XIAO reset target profile" against normal blind 1.8 separate body makes body 143 in component "REF XIAO"
ref_plane "WorkPlane1" through (0, 0, -20) normal (0, 0, 1) x (1, 0, 0) in component "REF DPDT"
sketch "DPDT body profile" plane through (0, 0, -20) normal (0, 0, 1) x (1, 0, 0) in component "REF DPDT"
  line L0 (55.7, 49.5) -> (64.3, 49.5)
  line L1 (64.3, 49.5) -> (64.3, 52.2)
  line L2 (64.3, 52.2) -> (55.7, 52.2)
  line L3 (55.7, 52.2) -> (55.7, 49.5)
  dimension "d1153" = 8.6
  dimension "d1154" = 2.7
  measures "d1153" horizontal distance of L0.start L0.end
  measures "d1154" vertical distance of L0.end L1.end
extrude "DPDT body" add sketch "DPDT body profile" against normal blind 3.1 separate body makes body 144 in component "REF DPDT"
ref_plane "WorkPlane2" through (0, 0, -20.84) normal (0, 0, 1) x (1, 0, 0) in component "REF DPDT"
sketch "DPDT actuator profile" plane through (0, 0, -20.84) normal (0, 0, 1) x (1, 0, 0) in component "REF DPDT"
  line L0 (59.29, 52.2) -> (60.71, 52.2)
  line L1 (60.71, 52.2) -> (60.71, 54.03)
  line L2 (60.71, 54.03) -> (59.29, 54.03)
  line L3 (59.29, 54.03) -> (59.29, 52.2)
  dimension "d1159" = 1.42
  dimension "d1160" = 1.83
  measures "d1159" horizontal distance of L0.start L0.end
  measures "d1160" vertical distance of L0.end L1.end
extrude "DPDT actuator" add sketch "DPDT actuator profile" against normal blind 1.42 separate body makes body 145 in component "REF DPDT"
ref_plane "WorkPlane3" through (0, 0, -20.4) normal (0, 0, 1) x (1, 0, 0) in component "REF DPDT"
sketch "DPDT terminal profile" plane through (0, 0, -20.4) normal (0, 0, 1) x (1, 0, 0) in component "REF DPDT"
  line L0 (56.8, 46.5) -> (57.2, 46.5)
  line L1 (57.2, 46.5) -> (57.2, 49.5)
  line L2 (57.2, 49.5) -> (56.8, 49.5)
  line L3 (56.8, 49.5) -> (56.8, 46.5)
  dimension "d1165" = 0.4
  dimension "d1166" = 3
  measures "d1165" horizontal distance of L0.start L0.end
  measures "d1166" vertical distance of L0.end L1.end
extrude "DPDT terminal" add sketch "DPDT terminal profile" against normal blind 0.35 separate body makes body 146 in component "REF DPDT"
ref_plane "WorkPlane4" through (0, 0, -22.2) normal (0, 0, 1) x (1, 0, 0) in component "REF DPDT"
sketch "DPDT terminal profile (1)" plane through (0, 0, -22.2) normal (0, 0, 1) x (1, 0, 0) in component "REF DPDT"
  line L0 (56.8, 46.5) -> (57.2, 46.5)
  line L1 (57.2, 46.5) -> (57.2, 49.5)
  line L2 (57.2, 49.5) -> (56.8, 49.5)
  line L3 (56.8, 49.5) -> (56.8, 46.5)
  dimension "d1171" = 0.4
  dimension "d1172" = 3
  measures "d1171" horizontal distance of L0.start L0.end
  measures "d1172" vertical distance of L0.end L1.end
extrude "DPDT terminal (1)" add sketch "DPDT terminal profile (1)" against normal blind 0.35 separate body makes body 147 in component "REF DPDT"
ref_plane "WorkPlane5" through (0, 0, -20.4) normal (0, 0, 1) x (1, 0, 0) in component "REF DPDT"
sketch "DPDT terminal profile (2)" plane through (0, 0, -20.4) normal (0, 0, 1) x (1, 0, 0) in component "REF DPDT"
  line L0 (59.8, 46.5) -> (60.2, 46.5)
  line L1 (60.2, 46.5) -> (60.2, 49.5)
  line L2 (60.2, 49.5) -> (59.8, 49.5)
  line L3 (59.8, 49.5) -> (59.8, 46.5)
  dimension "d1177" = 0.4
  dimension "d1178" = 3
  measures "d1177" horizontal distance of L0.start L0.end
  measures "d1178" vertical distance of L0.end L1.end
extrude "DPDT terminal (2)" add sketch "DPDT terminal profile (2)" against normal blind 0.35 separate body makes body 148 in component "REF DPDT"
ref_plane "WorkPlane6" through (0, 0, -22.2) normal (0, 0, 1) x (1, 0, 0) in component "REF DPDT"
sketch "DPDT terminal profile (3)" plane through (0, 0, -22.2) normal (0, 0, 1) x (1, 0, 0) in component "REF DPDT"
  line L0 (59.8, 46.5) -> (60.2, 46.5)
  line L1 (60.2, 46.5) -> (60.2, 49.5)
  line L2 (60.2, 49.5) -> (59.8, 49.5)
  line L3 (59.8, 49.5) -> (59.8, 46.5)
  dimension "d1183" = 0.4
  dimension "d1184" = 3
  measures "d1183" horizontal distance of L0.start L0.end
  measures "d1184" vertical distance of L0.end L1.end
extrude "DPDT terminal (3)" add sketch "DPDT terminal profile (3)" against normal blind 0.35 separate body makes body 149 in component "REF DPDT"
ref_plane "WorkPlane7" through (0, 0, -20.4) normal (0, 0, 1) x (1, 0, 0) in component "REF DPDT"
sketch "DPDT terminal profile (4)" plane through (0, 0, -20.4) normal (0, 0, 1) x (1, 0, 0) in component "REF DPDT"
  line L0 (62.8, 46.5) -> (63.2, 46.5)
  line L1 (63.2, 46.5) -> (63.2, 49.5)
  line L2 (63.2, 49.5) -> (62.8, 49.5)
  line L3 (62.8, 49.5) -> (62.8, 46.5)
  dimension "d1189" = 0.4
  dimension "d1190" = 3
  measures "d1189" horizontal distance of L0.start L0.end
  measures "d1190" vertical distance of L0.end L1.end
extrude "DPDT terminal (4)" add sketch "DPDT terminal profile (4)" against normal blind 0.35 separate body makes body 150 in component "REF DPDT"
ref_plane "WorkPlane8" through (0, 0, -22.2) normal (0, 0, 1) x (1, 0, 0) in component "REF DPDT"
sketch "DPDT terminal profile (5)" plane through (0, 0, -22.2) normal (0, 0, 1) x (1, 0, 0) in component "REF DPDT"
  line L0 (62.8, 46.5) -> (63.2, 46.5)
  line L1 (63.2, 46.5) -> (63.2, 49.5)
  line L2 (63.2, 49.5) -> (62.8, 49.5)
  line L3 (62.8, 49.5) -> (62.8, 46.5)
  dimension "d1195" = 0.4
  dimension "d1196" = 3
  measures "d1195" horizontal distance of L0.start L0.end
  measures "d1196" vertical distance of L0.end L1.end
extrude "DPDT terminal (5)" add sketch "DPDT terminal profile (5)" against normal blind 0.35 separate body makes body 151 in component "REF DPDT"
ref_plane "WorkPlane1" through (0, 0, -2.1875) normal (0, 0, 1) x (1, 0, 0) in component "REF Four LEDs"
sketch "LED module profile" plane through (0, 0, -2.1875) normal (0, 0, 1) x (1, 0, 0) in component "REF Four LEDs"
  line L0 (36, 2.8) -> (44, 2.8)
  line L1 (44, 2.8) -> (44, 10.8)
  line L2 (44, 10.8) -> (36, 10.8)
  line L3 (36, 10.8) -> (36, 2.8)
  dimension "d1201" = 8
  dimension "d1202" = 8
  measures "d1201" horizontal distance of L0.start L0.end
  measures "d1202" vertical distance of L0.end L1.end
extrude "LED module" add sketch "LED module profile" against normal blind 2 separate body makes body 152 in component "REF Four LEDs"
ref_plane "WorkPlane2" through (0, 0, -2.1875) normal (0, 0, 1) x (1, 0, 0) in component "REF Four LEDs"
sketch "LED module profile (1)" plane through (0, 0, -2.1875) normal (0, 0, 1) x (1, 0, 0) in component "REF Four LEDs"
  line L0 (36, 49.2) -> (44, 49.2)
  line L1 (44, 49.2) -> (44, 57.2)
  line L2 (44, 57.2) -> (36, 57.2)
  line L3 (36, 57.2) -> (36, 49.2)
  dimension "d1207" = 8
  dimension "d1208" = 8
  measures "d1207" horizontal distance of L0.start L0.end
  measures "d1208" vertical distance of L0.end L1.end
extrude "LED module (1)" add sketch "LED module profile (1)" against normal blind 2 separate body makes body 153 in component "REF Four LEDs"
ref_plane "WorkPlane3" through (0, 0, -2.1875) normal (0, 0, 1) x (1, 0, 0) in component "REF Four LEDs"
sketch "LED module profile (2)" plane through (0, 0, -2.1875) normal (0, 0, 1) x (1, 0, 0) in component "REF Four LEDs"
  line L0 (76, 2.8) -> (84, 2.8)
  line L1 (84, 2.8) -> (84, 10.8)
  line L2 (84, 10.8) -> (76, 10.8)
  line L3 (76, 10.8) -> (76, 2.8)
  dimension "d1213" = 8
  dimension "d1214" = 8
  measures "d1213" horizontal distance of L0.start L0.end
  measures "d1214" vertical distance of L0.end L1.end
extrude "LED module (2)" add sketch "LED module profile (2)" against normal blind 2 separate body makes body 154 in component "REF Four LEDs"
ref_plane "WorkPlane4" through (0, 0, -2.1875) normal (0, 0, 1) x (1, 0, 0) in component "REF Four LEDs"
sketch "LED module profile (3)" plane through (0, 0, -2.1875) normal (0, 0, 1) x (1, 0, 0) in component "REF Four LEDs"
  line L0 (76, 49.2) -> (84, 49.2)
  line L1 (84, 49.2) -> (84, 57.2)
  line L2 (84, 57.2) -> (76, 57.2)
  line L3 (76, 57.2) -> (76, 49.2)
  dimension "d1219" = 8
  dimension "d1220" = 8
  measures "d1219" horizontal distance of L0.start L0.end
  measures "d1220" vertical distance of L0.end L1.end
extrude "LED module (3)" add sketch "LED module profile (3)" against normal blind 2 separate body makes body 155 in component "REF Four LEDs"
ref_plane "WorkPlane1" through (0, 0, -0.2) normal (0, 0, 1) x (1, 0, 0) in component "REF M3 screws"
sketch "Closure screw head profile" plane through (0, 0, -0.2) normal (0, 0, 1) x (1, 0, 0) in component "REF M3 screws"
  circle A0 centre (6, 6) radius 2.75
  dimension "d1225" = 5.5
  measures "d1225" diameter of A0
extrude "Closure screw head" add sketch "Closure screw head profile" against normal blind 3 separate body makes body 156 in component "REF M3 screws"
ref_plane "WorkPlane2" through (0, 0, -3.2) normal (0, 0, 1) x (1, 0, 0) in component "REF M3 screws"
sketch "Closure screw shaft profile" plane through (0, 0, -3.2) normal (0, 0, 1) x (1, 0, 0) in component "REF M3 screws"
  circle A0 centre (6, 6) radius 1.5
  dimension "d1230" = 3
  measures "d1230" diameter of A0
extrude "Closure screw shaft" add sketch "Closure screw shaft profile" against normal blind 25 separate body makes body 157 in component "REF M3 screws"
ref_plane "WorkPlane3" through (0, 0, -0.2) normal (0, 0, 1) x (1, 0, 0) in component "REF M3 screws"
sketch "Closure screw head profile (1)" plane through (0, 0, -0.2) normal (0, 0, 1) x (1, 0, 0) in component "REF M3 screws"
  circle A0 centre (114, 6) radius 2.75
  dimension "d1235" = 5.5
  measures "d1235" diameter of A0
extrude "Closure screw head (1)" add sketch "Closure screw head profile (1)" against normal blind 3 separate body makes body 158 in component "REF M3 screws"
ref_plane "WorkPlane4" through (0, 0, -3.2) normal (0, 0, 1) x (1, 0, 0) in component "REF M3 screws"
sketch "Closure screw shaft profile (1)" plane through (0, 0, -3.2) normal (0, 0, 1) x (1, 0, 0) in component "REF M3 screws"
  circle A0 centre (114, 6) radius 1.5
  dimension "d1240" = 3
  measures "d1240" diameter of A0
extrude "Closure screw shaft (1)" add sketch "Closure screw shaft profile (1)" against normal blind 25 separate body makes body 159 in component "REF M3 screws"
ref_plane "WorkPlane5" through (0, 0, -0.2) normal (0, 0, 1) x (1, 0, 0) in component "REF M3 screws"
sketch "Closure screw head profile (2)" plane through (0, 0, -0.2) normal (0, 0, 1) x (1, 0, 0) in component "REF M3 screws"
  circle A0 centre (6, 54) radius 2.75
  dimension "d1245" = 5.5
  measures "d1245" diameter of A0
extrude "Closure screw head (2)" add sketch "Closure screw head profile (2)" against normal blind 3 separate body makes body 160 in component "REF M3 screws"
ref_plane "WorkPlane6" through (0, 0, -3.2) normal (0, 0, 1) x (1, 0, 0) in component "REF M3 screws"
sketch "Closure screw shaft profile (2)" plane through (0, 0, -3.2) normal (0, 0, 1) x (1, 0, 0) in component "REF M3 screws"
  circle A0 centre (6, 54) radius 1.5
  dimension "d1250" = 3
  measures "d1250" diameter of A0
extrude "Closure screw shaft (2)" add sketch "Closure screw shaft profile (2)" against normal blind 25 separate body makes body 161 in component "REF M3 screws"
ref_plane "WorkPlane7" through (0, 0, -0.2) normal (0, 0, 1) x (1, 0, 0) in component "REF M3 screws"
sketch "Closure screw head profile (3)" plane through (0, 0, -0.2) normal (0, 0, 1) x (1, 0, 0) in component "REF M3 screws"
  circle A0 centre (96, 54) radius 2.75
  dimension "d1255" = 5.5
  measures "d1255" diameter of A0
extrude "Closure screw head (3)" add sketch "Closure screw head profile (3)" against normal blind 3 separate body makes body 162 in component "REF M3 screws"
ref_plane "WorkPlane8" through (0, 0, -3.2) normal (0, 0, 1) x (1, 0, 0) in component "REF M3 screws"
sketch "Closure screw shaft profile (3)" plane through (0, 0, -3.2) normal (0, 0, 1) x (1, 0, 0) in component "REF M3 screws"
  circle A0 centre (96, 54) radius 1.5
  dimension "d1260" = 3
  measures "d1260" diameter of A0
extrude "Closure screw shaft (3)" add sketch "Closure screw shaft profile (3)" against normal blind 25 separate body makes body 163 in component "REF M3 screws"
ref_plane "WorkPlane9" through (0, 0, -9.075) normal (0, 0, 1) x (1, 0, 0) in component "REF M3 screws"
sketch "Optical screw head profile" plane through (0, 0, -9.075) normal (0, 0, 1) x (1, 0, 0) in component "REF M3 screws"
  circle A0 centre (60, 6) radius 2.85
  dimension "d1265" = 5.7
  measures "d1265" diameter of A0
extrude "Optical screw head" add sketch "Optical screw head profile" against normal blind 1.65 separate body makes body 164 in component "REF M3 screws"
ref_plane "WorkPlane10" through (0, 0, -3.075) normal (0, 0, 1) x (1, 0, 0) in component "REF M3 screws"
sketch "Optical screw shaft profile" plane through (0, 0, -3.075) normal (0, 0, 1) x (1, 0, 0) in component "REF M3 screws"
  circle A0 centre (60, 6) radius 1.5
  dimension "d1270" = 3
  measures "d1270" diameter of A0
extrude "Optical screw shaft" add sketch "Optical screw shaft profile" against normal blind 6 separate body makes body 165 in component "REF M3 screws"
ref_plane "WorkPlane11" through (0, 0, -9.075) normal (0, 0, 1) x (1, 0, 0) in component "REF M3 screws"
sketch "Optical screw head profile (1)" plane through (0, 0, -9.075) normal (0, 0, 1) x (1, 0, 0) in component "REF M3 screws"
  circle A0 centre (60, 54) radius 2.85
  dimension "d1275" = 5.7
  measures "d1275" diameter of A0
extrude "Optical screw head (1)" add sketch "Optical screw head profile (1)" against normal blind 1.65 separate body makes body 166 in component "REF M3 screws"